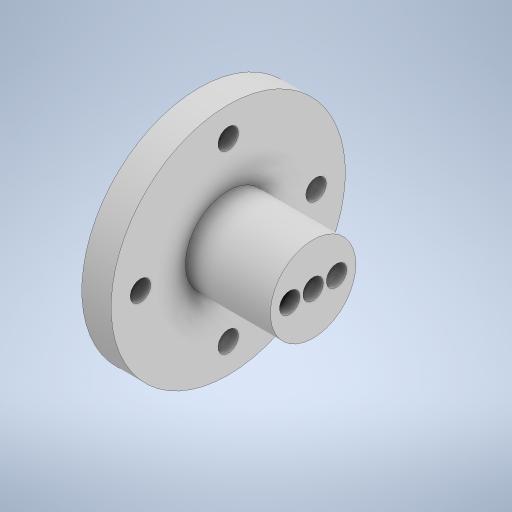
# Autodesk Inventor part: EaglePowerCycDriveAdaptor
Saved by Autodesk Inventor 2023 (Build 270158000, 158)
## iProperties
Created: 2023-03-29
Part Number: EaglePowerCycDriveAdaptor
Material: Generic
Document SubType Name: Sheet Metal
Designer: Charles Kelly
Density: 1 g/cm^3
Sheet Metal Rule: Default_mm
Appearance: Default
Author: Charles Kelly
Autodesk Inventor part; units mm, degrees
ref_plane "YZ Plane" through (0, 0, 0) normal (1, 0, 0) x (0, 1, 0)
ref_plane "XZ Plane" through (0, 0, 0) normal (0, 1, 0) x (-1, 0, 0)
ref_plane "XY Plane" through (0, 0, 0) normal (0, 0, 1) x (1, 0, 0)
sketch "Sketch1" plane through (0, 0, 0) normal (1, 0, 0) x (0, 1, 0)
  circle A0 centre (0, 0) radius 15
  circle A1 centre (15, 0) radius 1.75
  circle A2 centre (0, 15) radius 1.75
  circle A3 centre (-15, 0) radius 1.75
  circle A4 centre (0, -15) radius 1.75
  circle A5 centre (0, 0) radius 1.75
  circle A6 centre (0, 0) radius 20
  dimension "d0" = 30
  dimension "d1" = 3.5
  dimension "d4" = 360
  dimension "d6" = 3.5
  dimension "d7" = 40
  constraints: 6 centre point, 3 coincident, 1 horizontal alignment, 11 other
  measures "d1" diameter of A1
  measures "d6" diameter of A5
  measures "d7" diameter of A6
extrude "Extrusion1" add sketch "Sketch1" along normal blind 5 contours A1 A0 A4 A3 A2 | A6
sketch "Sketch5" plane through (5, 0, 0) normal (1, 0, 0) x (0, 0, -1)
  circle A0 centre (0, 0) radius 1.75 projected
  circle A1 centre (0, 0) radius 4
  circle A2 centre (4, 0) radius 1.75
  circle A3 centre (-4, 0) radius 1.75
  circle A4 centre (0, 0) radius 7.3
  dimension "d38" = 8
  dimension "d39" = 3.5
  dimension "d42" = 360
  dimension "d44" = 14.6
  constraints: 3 centre point, 2 coincident, 1 horizontal alignment, 7 other
  measures "d39" diameter of A2
  measures "d44" diameter of A4
extrude "Extrusion5" add sketch "Sketch5" along normal blind 14.5 contours A2 A1 A3 | A4
equation "\"BendRadius\" = Thickness"
equation "\"BendReliefWidth\" = Thickness"
equation "\"BendReliefDepth\" = 0.5 * Thickness"
equation "\"CornerReliefSize\" = 4 * Thickness"
equation "\"MinimumRemnant\" = 2 * Thickness"
equation "\"TransitionRadius\" = BendRadius"
equation "\"JacobiRadiusSize\" = BendRadius"
equation "\"GapSize\" = Thickness"
equation "\"Thickness\" = 0.5"
body "Solid1"
